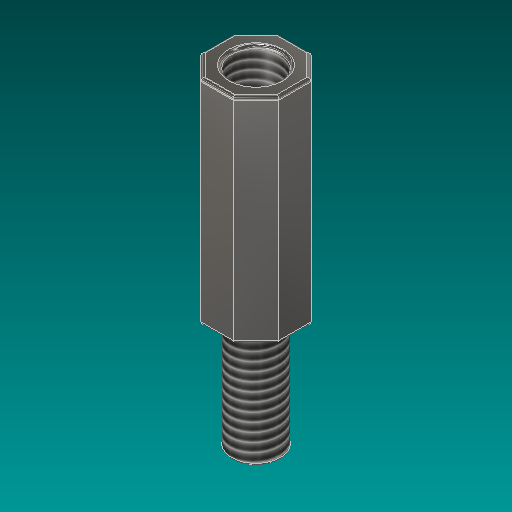
# Autodesk Inventor part: 11mm M2.5 standoff
Saved by Autodesk Inventor 2017 (Build 210142000, 142)
## iProperties
Created: 2016-07-05
Part Number: 11mm M2.5 standoff
Material: Steel, High Strength, Low Alloy
Document SubType Name: Modeling
Designer: Jonathan
Density: 7.85 g/cm^3
Appearance: Steel - Polished
Author: Jonathan
Autodesk Inventor part; units mm, degrees
ref_plane "YZ Plane" through (0, 0, 0) normal (1, 0, 0) x (0, 1, 0)
ref_plane "XZ Plane" through (0, 0, 0) normal (0, 1, 0) x (-1, 0, 0)
ref_plane "XY Plane" through (0, 0, 0) normal (0, 0, 1) x (1, 0, 0)
sketch "Sketch1" plane through (0, 0, 0) normal (0, 1, 0) x (-1, 0, 0)
  line L0 (0.8284, -2) -> (-0.8284, -2)
  line L1 (-0.8284, -2) -> (-2, -0.8284)
  line L2 (-2, -0.8284) -> (-2, 0.8284)
  line L3 (-2, 0.8284) -> (-0.8284, 2)
  line L4 (-0.8284, 2) -> (0.8284, 2)
  line L5 (0.8284, 2) -> (2, 0.8284)
  line L6 (2, 0.8284) -> (2, -0.8284)
  line L7 (2, -0.8284) -> (0.8284, -2)
  point P0 (0, 0)
  point P1 (0, -2)
  point P2 (2, 0)
  dimension "d1" = 135
  dimension "d2" = 4
  constraints: 16 end point, 5 equal length, 4 perpendicular, 2 midpoint, 2 parallel, 1 horizontal, 1 horizontal alignment, 1 vertical alignment
  measures "d1" angle of L1 L0
  measures "d2" distance between parallel lines of L4 L0
extrude "Extrusion1" add sketch "Sketch1" along normal blind 11
sketch "Sketch2" plane through (0, 11, 0) normal (0, 1, 0) x (1, 0, 0)
  circle A0 centre (0, 0) radius 1.25
  dimension "d5" = 2.5
  constraints: 1 centre point, 1 coincident
  measures "d5" diameter of A0
extrude "Extrusion2" cut sketch "Sketch2" against normal blind 6.35
thread "Thread1" size "M2.5x0.45" class "6H" standard "ANSI Metric M Profile" full length
sketch "Sketch3" plane through (0, 0, 0) normal (0, -1, 0) x (1, 0, 0)
  circle A0 centre (0, 0) radius 1.25
  dimension "d10" = 2.5
  constraints: 1 centre point, 1 coincident
  measures "d10" diameter of A0
extrude "Extrusion3" add sketch "Sketch3" along normal blind 6
thread "Thread2" size "M2.5x0.45" class "6g" standard "ANSI Metric M Profile" full length
fillet "Fillet1" radius 0.15 16 edges at (1.4142, 11, 1.4142) (2, 11, 0) (1.4142, 11, -1.4142) (0, 11, -2) (-1.4142, 11, -1.4142) (-2, 11, 0) (-1.4142, 11, 1.4142) (0, 11, 2) (1.4142, 0, 1.4142) (0, 0, 2) (-1.4142, 0, 1.4142) (-2, 0, 0) (0, 0, -2) (1.4142, 0, -1.4142) (2, 0, 0) (-1.4142, 0, -1.4142)
fillet "Fillet2" radius 0.15 1 edges at (-1.25, -6, 0)
fillet "Fillet3" radius 0.15 1 edges at (-1.25, 11, 0)
body "Solid1"
